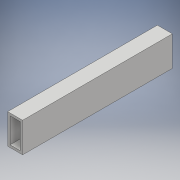
# Autodesk Inventor part: Pipe2
Saved by Autodesk Inventor 2018 (Build 220112000, 112)
## iProperties
Created: 2017-09-09
Part Number: Pipe2
Material: 一般
Document SubType Name: Modeling
Designer: mura5
Density: 1 g/cm^3
Appearance: 既定
Author: mura5
Autodesk Inventor part; units mm, degrees
ref_plane "YZ Plane" through (0, 0, 0) normal (1, 0, 0) x (0, 1, 0)
ref_plane "XZ Plane" through (0, 0, 0) normal (0, 1, 0) x (-1, 0, 0)
ref_plane "XY Plane" through (0, 0, 0) normal (0, 0, 1) x (1, 0, 0)
sketch "スケッチ2" plane through (0, 0, 0) normal (0, 1, 0) x (-1, 0, 0)
  line L0 (0, 0) -> (-20, 0)
  line L1 (-20, 0) -> (-20, 40)
  line L2 (-20, 40) -> (0, 40)
  line L3 (0, 40) -> (0, 0)
  line L4 (-3.2, 3.2) -> (-16.8, 3.2)
  line L5 (-16.8, 3.2) -> (-16.8, 36.8)
  line L6 (-16.8, 36.8) -> (-3.2, 36.8)
  line L7 (-3.2, 36.8) -> (-3.2, 3.2)
  dimension "d0" = 20
  dimension "d1" = 40
  dimension "d2" = 3.2
  constraints: 16 end point, 4 parallel, 2 perpendicular, 1 horizontal, 3 other
  measures "d0" distance of L1.end L2.end
  measures "d1" distance of L0.end L1.end
  measures "d2" distance between parallel lines of L3 L7
extrude "押し出し1" add sketch "スケッチ2" along normal blind 200
